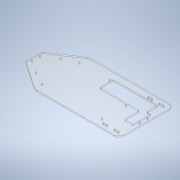
# Autodesk Inventor part: base
Saved by Autodesk Inventor 2020 (Build 240168000, 168)
## iProperties
Created: 2019-09-27
Part Number: base
Material: Polycarbonate, Clear
Document SubType Name: Modeling
Designer: n10208577
Density: 1.2 g/cm^3
Appearance: Polycarbonate - Clear
Author: n10208577
Autodesk Inventor part; units mm, degrees
ref_plane "YZ Plane" through (0, 0, 0) normal (1, 0, 0) x (0, 1, 0)
ref_plane "XZ Plane" through (0, 0, 0) normal (0, 1, 0) x (-1, 0, 0)
ref_plane "XY Plane" through (0, 0, 0) normal (0, 0, 1) x (1, 0, 0)
sketch "Sketch1" plane through (0, 0, 0) normal (0, 1, 0) x (-1, 0, 0)
  line L0 (-4.785, 96.1722) -> (-4.785, 46.1722)
  line L1 (176.1132, 106.1722) -> (5.215, 106.1722)
  line L2 (241.5136, 65.0993) -> (184.509, 103.6024)
  line L3 (-4.785, 46.1722) -> (-4.785, -3.8278)
  circle A0 centre (211.215, 73.1722) radius 1.6
  circle A1 centre (211.215, 19.1722) radius 1.6
  circle A2 centre (238.715, 54.9222) radius 1.6
  circle A3 centre (238.715, 37.4222) radius 1.6
  circle A4 centre (1.815, 37.7722) radius 1.6
  circle A5 centre (1.815, 54.5722) radius 1.6
  line L4 (243.715, 31.3885) -> (243.715, 60.9559)
  arc A6 (-4.785, -3.8278) -> (5.215, -13.8278) centre (5.215, -3.8278) ccw
  arc A7 (5.215, 106.1722) -> (-4.785, 96.1722) centre (5.215, 96.1722) ccw
  arc A8 (184.509, 103.6024) -> (176.1132, 106.1722) centre (176.1132, 91.1722) ccw
  arc A9 (176.1132, -13.8278) -> (184.509, -11.258) centre (176.1132, 1.1722) ccw
  arc A10 (243.715, 60.9559) -> (241.5136, 65.0993) centre (238.715, 60.9559) ccw
  arc A11 (241.5136, 27.2451) -> (243.715, 31.3885) centre (238.715, 31.3885) ccw
  line L5 (5.215, -13.8278) -> (176.1132, -13.8278)
  line L6 (184.509, -11.258) -> (241.5136, 27.2451)
  line L7 (5.215, 46.1722) -> (5.215, 64.1722)
  line L8 (6.215, 65.1722) -> (22.215, 65.1722)
  arc A12 (24.215, 63.1722) -> (22.215, 65.1722) centre (22.215, 63.1722) ccw
  arc A13 (6.215, 65.1722) -> (5.215, 64.1722) centre (6.215, 64.1722) ccw
  line L9 (24.215, 63.1722) -> (24.215, 34.1722)
  line L10 (12.215, 27.1722) -> (6.215, 27.1722)
  arc A14 (5.215, 28.1722) -> (6.215, 27.1722) centre (6.215, 28.1722) ccw
  line L11 (5.215, 28.1722) -> (5.215, 46.1722)
  line L12 (112.215, 30.1722) -> (112.215, 4.1722)
  arc A15 (110.215, 2.1722) -> (112.215, 4.1722) centre (110.215, 4.1722) ccw
  line L13 (110.215, 32.1722) -> (26.215, 32.1722)
  arc A16 (112.215, 30.1722) -> (110.215, 32.1722) centre (110.215, 30.1722) ccw
  arc A17 (24.215, 34.1722) -> (26.215, 32.1722) centre (26.215, 34.1722) ccw
  line L14 (110.215, 2.1722) -> (16.215, 2.1722)
  arc A18 (14.215, 4.1722) -> (16.215, 2.1722) centre (16.215, 4.1722) ccw
  line L15 (14.215, 4.1722) -> (14.215, 25.1722)
  arc A19 (14.215, 25.1722) -> (12.215, 27.1722) centre (12.215, 25.1722) ccw
  line L16 (41.565, -1.9278) -> (31.865, -1.9278)
  line L17 (31.865, -1.9278) -> (31.865, -4.7278)
  line L18 (36.715, -4.7278) -> (41.565, -4.7278)
  line L19 (41.565, -4.7278) -> (41.565, -1.9278)
  line L20 (36.715, -4.7278) -> (31.865, -4.7278)
  line L21 (16.565, -1.9278) -> (6.865, -1.9278)
  line L22 (6.865, -1.9278) -> (6.865, -4.7278)
  line L23 (11.715, -4.7278) -> (16.565, -4.7278)
  line L24 (16.565, -4.7278) -> (16.565, -1.9278)
  line L25 (11.715, -4.7278) -> (6.865, -4.7278)
  line L26 (41.565, 94.2722) -> (31.865, 94.2722)
  line L27 (31.865, 94.2722) -> (31.865, 97.0722)
  line L28 (36.715, 97.0722) -> (41.565, 97.0722)
  line L29 (41.565, 97.0722) -> (41.565, 94.2722)
  line L30 (36.715, 97.0722) -> (31.865, 97.0722)
  line L31 (16.565, 94.2722) -> (6.865, 94.2722)
  line L32 (6.865, 94.2722) -> (6.865, 97.0722)
  line L33 (11.715, 97.0722) -> (16.565, 97.0722)
  line L34 (16.565, 97.0722) -> (16.565, 94.2722)
  line L35 (11.715, 97.0722) -> (6.865, 97.0722)
  circle A20 centre (50.715, 36.1722) radius 1.6
  circle A21 centre (50.715, 88.1722) radius 1.6
  circle A22 centre (182.715, 88.1722) radius 1.6
  circle A23 centre (116.215, 6.1722) radius 1.6
  circle A24 centre (182.715, 6.1722) radius 1.6
  point P0 (0, 0)
  constraints: 72 end point, 28 point on circle, 25 centre point
extrude "Extrusion1" add sketch "Sketch1" along normal blind 3
body "Solid1"
